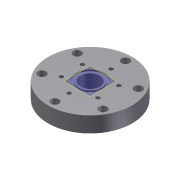
# Autodesk Inventor part: Conflat Flange
Saved by Autodesk Inventor 2011 (Build 150239000, 239)
## iProperties
Created: 2011-05-26
Part Number: Conflat Flange
Document SubType Name: Modeling
Designer: ijs09
Density: 1 g/cm^3
Author: ijs09
Autodesk Inventor part; units mm, degrees
ref_plane "YZ Plane" through (0, 0, 0) normal (1, 0, 0) x (0, 1, 0)
ref_plane "XZ Plane" through (0, 0, 0) normal (0, 1, 0) x (-1, 0, 0)
ref_plane "XY Plane" through (0, 0, 0) normal (0, 0, 1) x (1, 0, 0)
sketch "Sketch5" plane through (0, 0, 0) normal (0, 1, 0) x (-1, 0, 0)
  line L0 (-22.5, 13) -> (22.5, 13) construction
  line L1 (8, 13) -> (8, 0)
  line L2 (8, 0) -> (34.925, 0)
  line L3 (34.925, 0) -> (34.925, 13)
  line L4 (34.925, 13) -> (11.9, 13)
  line L5 (11.9, 11.8) -> (9.5, 11.8)
  line L6 (9.5, 11.8) -> (9.5, 13)
  line L7 (11.9, 11.8) -> (11.9, 13)
  line L8 (0, -1.501) -> (0, 14.3549) construction
  line L9 (8, 13) -> (9.5, 13)
  dimension "d38" = 13
  dimension "d39" = 8
  dimension "d40" = 9.5
  dimension "d41" = 2.4
  dimension "d42" = 1.2
  dimension "d43" = 34.925
  constraints: 20 end point, 4 parallel, 3 perpendicular, 3 point on line, 2 collinear, 1 horizontal, 1 vertical, 2 other
  measures "d38" distance between parallel lines of L2 L0
  measures "d39" distance between parallel lines of L1 L8
  measures "d40" distance between parallel lines of L6 L8
  measures "d41" distance between parallel lines of L7 L6
  measures "d42" distance between parallel lines of L0 L5
  measures "d43" distance between parallel lines of L8 L3
ref_plane "Work Plane1" through (0, 0, 13) normal (0, 0, -1) x (-1, 0, 0)
revolve "Revolution1" add sketch "Sketch5" angle 360 about axis through (0, 0, -1.501) along (0, 0, 1)
sketch "Sketch9" plane through (0, 0, 13) normal (0, 0, 1) x (1, 0, 0)
  circle A0 centre (0, 0) radius 11.9 projected
  circle A1 centre (0, 0) radius 17.5
  circle A2 centre (0, 0) radius 17.5
  circle A3 centre (0, 0) radius 17.5
  circle A4 centre (0, 0) radius 17.5
  circle A5 centre (0, 0) radius 17.5
  circle A6 centre (0, 0) radius 17.5
  point P0 (0, 17.5)
  point P1 (-15.1554, 8.75)
  point P2 (-15.1554, -8.75)
  point P3 (0, -17.5)
  point P4 (15.1554, -8.75)
  point P5 (15.1554, 8.75)
  dimension "d75" = 35
  dimension "d78" = 360
  constraints: 3 coincident, 2 vertical alignment, 33 other
hole "Hole6" at (0, 17.5, 13) at (-15.1554, 8.75, 13) at (-15.1554, -8.75, 13) at (0, -17.5, 13) at (15.1554, -8.75, 13) at (15.1554, 8.75, 13) direction (0, 0, -1) diameter 3.242 depth 7 tip angle 118 thread size "M4x0.7" class "6H" standard "ISO Metric profile"
sketch "Sketch10" plane through (0, 0, 13) normal (0, 0, 1) x (1, 0, 0)
  circle A0 centre (0, 0) radius 11.9 projected
  circle A1 centre (0, 0) radius 29.35
  point P0 (0, 29.35)
  point P1 (-25.4178, 14.675)
  point P2 (-25.4178, -14.675)
  point P3 (0, -29.35)
  point P4 (25.4178, -14.675)
  point P5 (25.4178, 14.675)
  dimension "d87" = 58.7
  dimension "d90" = 360
  constraints: 1 coincident, 1 vertical alignment, 9 other
hole "Hole7" at (0, 29.35, 13) at (-25.4178, 14.675, 13) at (-25.4178, -14.675, 13) at (0, -29.35, 13) at (25.4178, -14.675, 13) at (25.4178, 14.675, 13) direction (0, 0, -1) diameter 6.7 end through all
body "Solid2"
